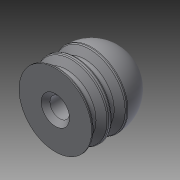
# Autodesk Inventor part: VertebraeSimple
Saved by Autodesk Inventor 2014 SP1 (Build 180222100, 222)
## iProperties
Created: 2014-11-10
Part Number: VertebraeSimple
Material: Generic
Document SubType Name: Modeling
Designer: rawrdong
Density: 1 g/cm^3
Appearance: Default
Author: rawrdong
Autodesk Inventor part; units mm, degrees
ref_plane "YZ Plane" through (0, 0, 0) normal (1, 0, 0) x (0, 1, 0)
ref_plane "XZ Plane" through (0, 0, 0) normal (0, 1, 0) x (-1, 0, 0)
ref_plane "XY Plane" through (0, 0, 0) normal (0, 0, 1) x (1, 0, 0)
sketch "Sketch1" plane through (0, 0, 0) normal (0, 0, 1) x (1, 0, 0)
  arc A0 (12.5, 0) -> (3.375, 12.0358) centre (0, 0) ccw
  line L0 (12.5, 0) -> (3.375, 0) construction
  line L1 (3.375, 0) -> (3.375, 12.0358)
  line L2 (0, -17.714) -> (0, 18.7837) construction
  line L3 (3.375, 0) -> (3.375, -12.5)
  line L4 (3.375, -12.5) -> (12.5, -12.5)
  line L5 (12.5, -11.8981) -> (8.8966, -9.375)
  line L6 (8.8966, -9.375) -> (12.5, -6.8519)
  line L7 (3.375, -6.25) -> (12.5, -6.25)
  line L8 (12.5, -0.6019) -> (8.8966, -3.125)
  line L9 (8.8966, -3.125) -> (12.5, -5.6481)
  line L10 (12.5, -12.5) -> (12.5, -11.8981)
  line L11 (12.5, -6.8519) -> (12.5, -5.6481)
  line L12 (12.5, -0.6019) -> (12.5, 0)
  line L13 (8.8966, -9.375) -> (8.8966, -6.25) construction
  line L14 (8.8966, -9.375) -> (8.8966, -12.5) construction
  dimension "d1" = 3.375
  dimension "d6" = 12.5
  dimension "d7" = 12.5
  dimension "d9" = 35
  dimension "d10" = 35
  constraints: 28 end point, 5 parallel, 4 symmetric about line, 3 coincident, 3 perpendicular, 3 point on line, 3 tangent, 2 midpoint, 2 point on circle, 1 centre point, 1 collinear, 1 horizontal, 2 other
  measures "d1" distance between parallel lines of L1 L2
  measures "d6" radius of A0
  measures "d7" distance of L4.end L0.start
  measures "d9" angle of L4 L5
  measures "d10" angle of L0 L6
revolve "Revolution1" add sketch "Sketch1" angle 360 about axis through (0, -10, 0) along (0, 1, 0)
chamfer "Chamfer1" distance 1.5 angle 45 1 edges at (-3.375, -12.5, 0)
fillet "Fillet1" radius 1.5 1 edges at (-3.375, 12.0358, 0)
fillet "Fillet2" radius 1 2 edges at (-8.8966, -3.125, 0) (-8.8966, -9.375, 0)
fillet "Fillet3" radius 0.5 4 edges at (-12.5, -0.6019, 0) (-12.5, -5.6481, 0) (-12.5, -6.8519, 0) (-12.5, -11.8981, 0)
body "Solid1"
